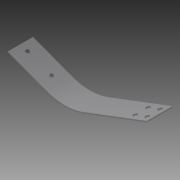
# Autodesk Inventor part: ski poly
Saved by Autodesk Inventor 2014 SP1 (Build 180222100, 222)
## iProperties
Created: 2013-10-24
Part Number: ski poly
Material: Polycarbonate, Clear
Document SubType Name: Modeling
Designer: RyanHughes
Density: 1.2 g/cm^3
Appearance: Polycarbonate - Clear
Author: RyanHughes
Autodesk Inventor part; units mm, degrees
ref_plane "YZ Plane" through (0, 0, 0) normal (1, 0, 0) x (0, 1, 0)
ref_plane "XZ Plane" through (0, 0, 0) normal (0, 1, 0) x (-1, 0, 0)
ref_plane "XY Plane" through (0, 0, 0) normal (0, 0, 1) x (1, 0, 0)
sketch "Sketch1" plane through (0, 0, 0) normal (0, 1, 0) x (-1, 0, 0)
  line L0 (88.9, -12.7) -> (-88.9, -12.7)
  line L1 (-88.9, -12.7) -> (-88.9, 12.7)
  line L2 (-88.9, 12.7) -> (88.9, 12.7)
  line L3 (88.9, 12.7) -> (88.9, -12.7)
  line L4 (88.9, -12.7) -> (-88.9, 12.7) construction
  line L5 (-88.9, -12.7) -> (88.9, 12.7) construction
  point P0 (0, 0)
  dimension "d0" = 177.8
  dimension "d1" = 25.4
  constraints: 12 end point, 2 midpoint, 2 parallel, 1 horizontal, 1 perpendicular
  measures "d0" distance of L1.end L2.end
  measures "d1" distance of L0.end L1.end
extrude "Extrusion1" add sketch "Sketch1" along normal blind 1.5875
sketch "Sketch2" plane through (0, 1.5875, 0) normal (0, 1, 0) x (1, 0, 0)
  line L0 (88.9, 12.7) -> (-88.9, 12.7) projected
  line L1 (88.9, -12.7) -> (88.9, 12.7) projected
  circle A0 centre (82.55, 6.35) radius 1.905
  circle A1 centre (69.85, 6.35) radius 1.905
  circle A2 centre (82.55, -6.35) radius 1.905
  circle A3 centre (69.85, -6.35) radius 1.905
  point P0 (0, 0)
  dimension "d6" = 3.81
  dimension "d7" = 6.35
  dimension "d8" = 6.35
  dimension "d11" = 12.7
  dimension "d14" = 12.7
  constraints: 4 centre point, 1 horizontal, 1 vertical, 6 other
  measures "d6" diameter of A0
  measures "d7" distance from line of L1 A0.centre
  measures "d8" distance from line of L0 A0.centre
  measures "d11" distance of A0.centre A1.centre
  measures "d14" distance of A0.centre A2.centre
extrude "Extrusion2" cut sketch "Sketch2" against normal blind 1.5875
sketch "Sketch3" plane through (0, 1.5875, 0) normal (0, 1, 0) x (1, 0, 0)
  line L0 (-88.9, 12.7) -> (-88.9, -12.7) projected
  line L1 (88.9, -12.7) -> (88.9, 12.7) projected
  line L2 (2.54, 28.0863) -> (2.54, -27.7339)
  point P0 (0, 0)
  dimension "d20" = 86.36
  constraints: 2 end point, 1 parallel
  measures "d20" distance between parallel lines of L1 L2
bend part "Bend Part1" radius 50.8 angle 41.47 line through (2.54, 1.5875, -28.0863) along (0, 0, 1) centre toward (0, 1, 0) moving side (1, 0, 0) both sides yes
sketch "Sketch4" plane through (-15.4455, 4.8779, 12.7) normal (0.3540462, 0.9352279, 0) x (0.9352279, -0.3540462, 0)
  line L0 (-73.0558, 25.4) -> (-73.0558, 0) projected
  line L1 (-91.9102, 34.6791) -> (-41.3058, 34.6791)
  line L2 (-41.3058, 34.6791) -> (-41.3058, -12.5805)
  line L3 (-41.3058, -12.5805) -> (-91.9102, -12.5805)
  line L4 (-91.9102, -12.5805) -> (-91.9102, 34.6791)
  point P0 (16.1721, 12.7)
  dimension "d23" = 31.75
  constraints: 8 end point, 2 parallel, 1 horizontal, 1 perpendicular
  measures "d23" distance between parallel lines of L0 L2
extrude "Extrusion3" cut sketch "Sketch4" against normal blind 1.5875
sketch "Sketch5" plane through (-15.4455, 4.8779, 12.7) normal (0.3540462, 0.9352279, 0) x (0.9352279, -0.3540462, 0)
  line L0 (-41.3058, 25.4) -> (-41.3058, 0) projected
  line L1 (0, 25.4) -> (-41.3058, 25.4) projected
  circle A0 centre (-33.635, 12.7) radius 1.905
  circle A1 centre (-8.235, 12.7) radius 1.905
  point P0 (16.1721, 12.7)
  dimension "d26" = 3.81
  dimension "d27" = 7.6708
  dimension "d28" = 12.7
  dimension "d31" = 25.4
  constraints: 2 centre point, 1 horizontal, 2 other
  measures "d26" diameter of A0
  measures "d27" distance from line of L0 A0.centre
  measures "d28" distance from line of A0.centre L1
  measures "d31" distance of A0.centre A1.centre
extrude "Extrusion4" cut sketch "Sketch5" against normal blind 1.5875
fillet "Fillet1" radius 0.508 18 edges at (-54.0759, 19.5021, 0) (-34.7607, 12.19, 12.7) (-34.7607, 12.19, -12.7) (2.54, 1.5875, 12.7) (52.312, 16.9112, 12.7) (2.54, 1.5875, -12.7) (52.312, 16.9112, -12.7) (2.54, 0, -12.7) (2.54, 0, 12.7) (52.874, 15.4265, -12.7) (-35.3228, 10.7053, -12.7) (-35.3228, 10.7053, 12.7) (52.874, 15.4265, 12.7) (84.3794, 28.2022, 12.7) (84.3794, 28.2022, -12.7) (84.0984, 28.9445, 0) (84.6604, 27.4598, 0) (-54.6379, 18.0174, 0)
body "Solid1"
